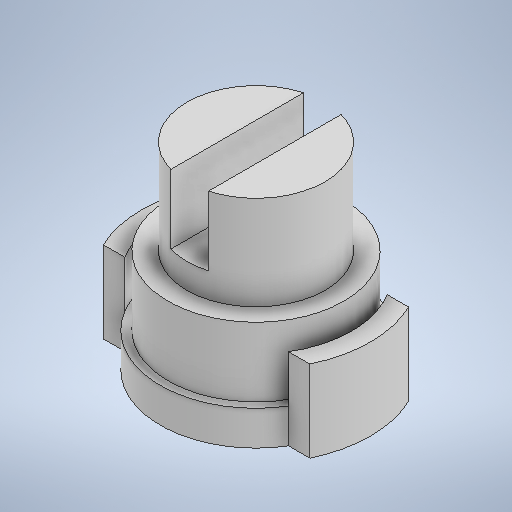
# Autodesk Inventor part: Light Water Sensor
Saved by Autodesk Inventor 2025 (Build 290162000, 162)
## iProperties
Created: 2024-07-09
Part Number: Light Water Sensor
Material: Generic
Document SubType Name: Modeling
Designer: track
Density: 1 g/cm^3
Appearance: Default
Author: track
Autodesk Inventor part; units mm, degrees
ref_plane "YZ Plane" through (0, 0, 0) normal (1, 0, 0) x (0, 1, 0)
ref_plane "XZ Plane" through (0, 0, 0) normal (0, 1, 0) x (-1, 0, 0)
ref_plane "XY Plane" through (0, 0, 0) normal (0, 0, 1) x (1, 0, 0)
sketch "Sketch1" plane through (0, 0, 0) normal (0, 1, 0) x (-1, 0, 0)
  circle A0 centre (0, 0) radius 14
  dimension "d0" = 28
  constraints: 1 centre point, 1 coincident
  measures "d0" diameter of A0
extrude "Extrusion1" add sketch "Sketch1" along normal blind 16.5
sketch "Sketch2" plane through (0, 16.5, 0) normal (0, 1, 0) x (1, 0, 0)
  circle A0 centre (0, 0) radius 11
  dimension "d3" = 22
  constraints: 1 centre point, 1 coincident
  measures "d3" diameter of A0
extrude "Extrusion2" add sketch "Sketch2" along normal blind 15
sketch "Sketch3" plane through (0, 31.5, 0) normal (0, 1, 0) x (1, 0, 0)
  line L0 (-3, -11) -> (3, -11)
  line L1 (3, -11) -> (3, 11)
  line L2 (3, 11) -> (-3, 11)
  line L3 (-3, 11) -> (-3, -11)
  line L4 (-3, -11) -> (3, 11) construction
  line L5 (3, -11) -> (-3, 11) construction
  circle A0 centre (0, 0) radius 11 projected
  point P0 (3, -10.583)
  point P1 (3, 10.583)
  point P2 (-3, 10.583)
  point P3 (-3, -10.583)
  dimension "d6" = 6
  dimension "d7" = 0
  constraints: 12 end point, 2 midpoint, 2 parallel, 1 horizontal, 1 perpendicular
  measures "d6" distance of L1.end L2.end
  measures "d7" distance edge to line of A0 L2
extrude "Extrusion3" cut sketch "Sketch3" against normal blind 11 contours A0 L3 L1
sketch "Sketch4" plane through (0, 0, 0) normal (0, -1, 0) x (1, 0, 0)
  circle A0 centre (0, 0) radius 15.25
  dimension "d10" = 30.5
  constraints: 1 centre point, 1 coincident
  measures "d10" diameter of A0
extrude "Extrusion4" add sketch "Sketch4" against normal blind 5.5
sketch "Sketch5" plane through (0, 0, 0) normal (0, -1, 0) x (1, 0, 0)
  line L0 (-16.4635, -7.875) -> (16.4635, -7.875)
  line L1 (16.4635, 7.875) -> (-16.4635, 7.875)
  circle A0 centre (0, 0) radius 15.25 projected
  arc A1 (-16.4635, 7.875) -> (-16.4635, -7.875) centre (0, 0) ccw
  arc A2 (16.4635, -7.875) -> (16.4635, 7.875) centre (0, 0) ccw
  point P0 (-13.0594, -7.875)
  point P1 (-13.0594, 7.875)
  point P2 (13.0594, 7.875)
  point P3 (13.0594, -7.875)
  dimension "d15" = 15.75
  dimension "d16" = 7.875
  dimension "d17" = 18.25
  dimension "d18" = 18.25
  dimension "d19" = 0
  constraints: 4 end point, 4 point on circle, 2 centre point, 1 horizontal, 1 parallel
  measures "d15" distance between parallel lines of L0 L1
  measures "d16" distance from line of point (0, 0) L1
  measures "d17" radius of A1
  measures "d18" radius of A2
  measures "d19" distance of point (0, 0) A1.centre
extrude "Extrusion5" add sketch "Sketch5" against normal blind 13 contours A1 L1 A0 L0 | A0 L1 A2 L0
body "Solid1"
